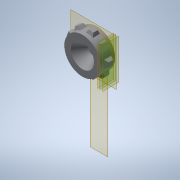
# Autodesk Inventor part: wheel_FRONT
Saved by Autodesk Inventor 2020 (Build 240168000, 168)
## iProperties
Created: 2020-04-12
Part Number: wheel_FRONT
Material: Ogólny
Document SubType Name: Modeling
Designer: blep
Density: 1 g/cm^3
Appearance: Domyślna
Author: blep
Autodesk Inventor part; units mm, degrees
ref_plane "YZ Plane" through (0, 0, 0) normal (1, 0, 0) x (0, 1, 0)
ref_plane "XZ Plane" through (0, 0, 0) normal (0, 1, 0) x (-1, 0, 0)
ref_plane "XY Plane" through (0, 0, 0) normal (0, 0, 1) x (1, 0, 0)
ref_plane "Płaszczyzna konstrukcyjna1" through (-6.2, -86.5, 1) normal (0, 0, 1) x (0, -1, 0)
sketch "Szkic1" plane through (-6.2, -86.5, 1) normal (0, 0, 1) x (0, -1, 0)
  arc A0 (-86.6773, 8.9692) -> (-86.6773, 3.4308) centre (-92, 6.2) ccw construction
  circle A1 centre (-92, 6.2) radius 10
  circle A2 centre (-92, 6.2) radius 25
  point P0 (-86.5, 6.2)
  dimension "d0" = 20
  dimension "d1" = 50
  constraints: 2 centre point, 2 coincident
  measures "d0" diameter of A1
  measures "d1" diameter of A2
extrude "Wyciągnięcie proste1" add sketch "Szkic1" along normal blind 20
ref_plane "Płaszczyzna konstrukcyjna2" through (0, 4.593, 6) normal (0, 0, 1) x (1, 0, 0)
sketch "Szkic3" plane through (0, 5.5, 21) normal (0, 0, 1) x (1, 0, 0)
  circle A0 centre (0, 0) radius 10 projected
  point P0 (0, -5.5)
extrude "Wyciągnięcie proste2" add sketch "Szkic3" against normal up to surface (20 mm away)
sketch "Szkic4" plane through (0, 5.5, 21) normal (0, 0, 1) x (1, 0, 0)
  circle A0 centre (0, 0) radius 25 construction
  circle A1 centre (0, 0) radius 2.125
  point P0 (0, -5.5)
  dimension "d6" = 4.25
  constraints: 1 centre point, 1 coincident
  measures "d6" diameter of A1
extrude "Wyciągnięcie proste3" cut sketch "Szkic4" against normal through all
ref_plane "Płaszczyzna konstrukcyjna4" through (25, 5.5, 1) normal (-1, 0, 0) x (0, -1, 0)
ref_plane "Płaszczyzna konstrukcyjna3" through (-8.2, -33.5, -38) normal (-1, 0, 0) x (0, 1, 0)
ref_plane "Płaszczyzna konstrukcyjna5" through (22, 5.5, 1) normal (-1, 0, 0) x (0, -1, 0)
sketch "Szkic5" plane through (22, 5.5, 1) normal (-1, 0, 0) x (0, -1, 0)
  line L0 (25, 0) -> (-25, 0) construction
  line L1 (25, 20) -> (-25, 20) construction
  line L2 (-25, 0) -> (-25, 20) construction
  line L3 (25, 0) -> (25, 20) construction
  line L4 (-6, 4) -> (6, 4)
  line L5 (6, 4) -> (6, 16)
  line L6 (6, 16) -> (-6, 16)
  line L7 (-6, 16) -> (-6, 4)
  line L8 (-6, 4) -> (-6, 0) construction
  line L9 (-6, 16) -> (-6, 20) construction
  line L10 (-6, 16) -> (-25, 16) construction
  line L11 (6, 16) -> (25, 16) construction
  point P0 (5.5, -1)
  dimension "d10" = 12
  dimension "d11" = 12
  constraints: 16 end point, 4 point on line, 3 horizontal, 2 collinear, 2 parallel, 2 vertical, 1 perpendicular
  measures "d10" distance of L4.end L5.end
  measures "d11" distance of L5.end L6.end
ref_plane "Płaszczyzna konstrukcyjna6" through (29, 5.5, 1) normal (-1, 0, 0) x (0, -1, 0)
sketch "Szkic6" plane through (29, 5.5, 1) normal (-1, 0, 0) x (0, -1, 0)
  line L0 (-6, 4) -> (6, 4) construction
  line L1 (6, 16) -> (-6, 16) construction
  line L2 (-6, 16) -> (-6, 4) construction
  line L3 (6, 4) -> (6, 16) construction
  line L4 (3, 7) -> (-3, 7)
  line L5 (-3, 7) -> (-3, 13)
  line L6 (-3, 13) -> (3, 13)
  line L7 (3, 13) -> (3, 7)
  point P0 (5.5, -1)
  dimension "d13" = 3
  constraints: 8 end point, 3 other
  measures "d13" distance between parallel lines of L0 L4
loft "Wyciągnięcie złożone1" add profiles "Szkic5", "Szkic6"
pattern_circular "Szyk kołowy1" count 9 over 360 about axis through (0, 5.5, 21) along (0, 0, -1) of "Wyciągnięcie złożone1"
sketch "Szkic7" plane through (0, 5.5, 21) normal (0, 0, 1) x (1, 0, 0)
  circle A0 centre (0, 0) radius 6
  point P0 (0, -5.5)
  dimension "d24" = 12
  constraints: 1 centre point
  measures "d24" diameter of A0
extrude "Wyciągnięcie proste4" cut sketch "Szkic7" against normal blind 14
chamfer "Faza2" distance 10 distance2 14 1 edges at (-6, 5.5, 21) measured on face at (-6.5, 5.5, 21)
